Autodesk Inventor part; units mm, degrees
(part 2 of 2)
sketch "Sketch11" plane through (0, 30, 0) normal (0, 1, 0) x (1, 0, 0)
  circle A0 centre (-41.8579, 41.8579) radius 1.925 construction
  arc A1 (45.0398, -38.6759) -> (38.6759, -45.0398) centre (41.8579, -41.8579) ccw construction
  line L0 (-41.8579, 41.8579) -> (41.8579, -41.8579) construction
  circle A2 centre (-41.8579, -41.8579) radius 1.925 construction
  circle A3 centre (41.8579, 41.8579) radius 1.925 construction
  line L1 (-41.8579, -41.8579) -> (41.8579, 41.8579) construction
  arc A4 (-45.0398, 38.6759) -> (-38.6759, 45.0398) centre (-41.8579, 41.8579) ccw construction
  line L2 (41.8579, 41.8579) -> (-41.8579, 41.8579) construction
  arc A5 (-38.6759, -45.0398) -> (-38.4709, -38.895) centre (-41.8579, -41.8579) ccw construction
  line L3 (-41.8579, 41.8579) -> (-41.8579, -41.8579) construction
  circle A6 centre (41.8579, -41.8579) radius 1.925 construction
  line L4 (-41.8579, -41.8579) -> (41.8579, -41.8579) construction
  line L5 (41.8579, -41.8579) -> (41.8579, 41.8579) construction
  point P0 (0, 0)
  constraints: 12 end point, 2 perpendicular, 1 horizontal
sketch "Sketch12" plane through (0, 3, 0) normal (0, 1, 0) x (1, 0, 0)
  circle A0 centre (-47.9582, 35.11) radius 4.5 projected
  line L0 (-47.9582, 30.61) -> (-53, 30.61)
  line L1 (-44.7763, 38.292) -> (-48.282, 41.7977)
  line L2 (-53, 37.0797) -> (-37.0797, 53) projected
  line L3 (-53, -37.0797) -> (-53, 37.0797) projected
  circle A1 centre (-47.9582, -7.09) radius 4.5 projected
  line L4 (-47.9582, -2.59) -> (-53, -2.59)
  line L5 (-47.9582, -11.59) -> (-53, -11.59)
  circle A2 centre (-47.8082, -33.0896) radius 4.5 projected
  line L6 (-47.8082, -28.5896) -> (-53, -28.5896)
  line L7 (-44.6263, -36.2715) -> (-49.2172, -40.8625)
  line L8 (-37.0797, -53) -> (-53, -37.0797) projected
  circle A3 centre (-47.8082, -33.0896) radius 4.5 projected
  line L9 (-37.0797, -53) -> (-53, -37.0797) projected
  point P0 (0, 0)
  constraints: 12 end point, 6 perpendicular, 6 point on line, 5 point on circle, 5 tangent, 2 horizontal, 2 other
extrude "Extrusion11" add sketch "Sketch12" along normal up to surface (8 mm away) contours L6 A2 L7 L8 L3 | L4 A1 L5 L3 | A0 L0 L3 L2 L1
body "Solid1"
